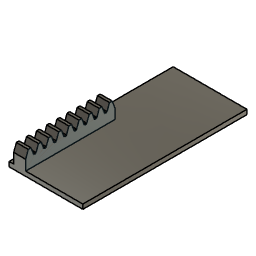
puerta mecatronica v1 (Autodesk Fusion 360 design; units mm, degrees)
Autodesk Fusion 360 part; units mm, degrees
sketch "Boceto1" plane through (0, 0, 0) normal (1, 0, 0) x (0, 1, 0)
  line L0 (0, 0) -> (1.5924, 4.375)
  line L1 (7.1092, 4.375) -> (8.7018, 0)
  line L2 (1.5924, 4.375) -> (2.8663, 7.875)
  line L3 (7.1092, 4.375) -> (5.8351, 7.875)
  line L4 (2.8663, 7.875) -> (5.8351, 7.875)
  line L5 (8.7018, 0) -> (0, 0)
  dimension "d8" = 4.375
  dimension "d9" = 3.5
  dimension "d10" = 3.5
  dimension "d11" = 4.375
  constraint coincident L0.start L5.end
  constraint parallel L0 L2
  constraint parallel L1 L3
  constraint horizontal L5
  measures "d8" vertical distance of L0.start L0.end
  measures "d9" vertical distance of L0.end L2.end
  measures "d10" vertical distance of L1.start L3.end
  measures "d11" vertical distance of L1.start L1.end
extrude "Extruir1" add sketch "Boceto1" along normal blind 13 makes body 1
pattern_linear "Patrón R1" count 9 spacing 11 along (0, -1, 0) of "Extruir1" makes body 2 makes body 3 makes body 4 makes body 5 makes body 6 makes body 7 makes body 8 makes body 9
sketch "Boceto2" plane through (13, 0, 0) normal (1, 0, 0) x (0, 1, 0)
  line L0 (8.7018, 0) -> (5.8351, 7.875)
  line L1 (5.8351, 7.875) -> (2.8663, 7.875)
  line L2 (2.8663, 7.875) -> (0, 0)
  line L3 (0, 0) -> (8.7018, 0)
  line L4 (-88, 0) -> (9, 0)
  line L5 (9, 0) -> (9, -16)
  line L6 (9, -16) -> (-88, -16)
  line L7 (-88, -16) -> (-88, 0)
  dimension "d18" = 16
  constraint horizontal L4
  constraint vertical L5
  constraint horizontal L6
  constraint vertical L7
  measures "d18" distance of L4.start L6.end
extrude "Extruir2" add sketch "Boceto2" against normal blind 13 contours L3 L4 L5 L6 L7 bodies 1 2 3 4 5 6 7 8 9
sketch "Boceto3" plane through (0, 0, 0) normal (-1, 0, 0) x (0, -1, 0)
  line L0 (71.1649, 7.875) -> (68.2982, 0)
  line L1 (68.2982, 0) -> (66, 0)
  line L2 (66, 0) -> (63.1337, 7.875)
  line L3 (63.1337, 7.875) -> (60.1649, 7.875)
  line L4 (60.1649, 7.875) -> (57.2982, 0)
  line L5 (57.2982, 0) -> (55, 0)
  line L6 (55, 0) -> (52.1337, 7.875)
  line L7 (52.1337, 7.875) -> (49.1649, 7.875)
  line L8 (49.1649, 7.875) -> (46.2982, 0)
  line L9 (46.2982, 0) -> (44, 0)
  line L10 (44, 0) -> (41.1337, 7.875)
  line L11 (41.1337, 7.875) -> (38.1649, 7.875)
  line L12 (38.1649, 7.875) -> (35.2982, 0)
  line L13 (35.2982, 0) -> (33, 0)
  line L14 (33, 0) -> (30.1337, 7.875)
  line L15 (30.1337, 7.875) -> (27.1649, 7.875)
  line L16 (27.1649, 7.875) -> (24.2982, 0)
  line L17 (24.2982, 0) -> (22, 0)
  line L18 (22, 0) -> (19.1337, 7.875)
  line L19 (19.1337, 7.875) -> (16.1649, 7.875)
  line L20 (16.1649, 7.875) -> (13.2982, 0)
  line L21 (13.2982, 0) -> (11, 0)
  line L22 (11, 0) -> (8.1337, 7.875)
  line L23 (8.1337, 7.875) -> (5.1649, 7.875)
  line L24 (5.1649, 7.875) -> (2.2982, 0)
  line L25 (2.2982, 0) -> (0, 0)
  line L26 (0, 0) -> (-2.8663, 7.875)
  line L27 (-2.8663, 7.875) -> (-5.8351, 7.875)
  line L28 (-5.8351, 7.875) -> (-8.7018, 0)
  line L29 (-8.7018, 0) -> (-9, 0)
  line L30 (-9, 0) -> (-9, -16)
  line L31 (-9, -16) -> (88, -16)
  line L32 (88, -16) -> (88, 0)
  line L33 (88, 0) -> (85.1337, 7.875)
  line L34 (85.1337, 7.875) -> (82.1649, 7.875)
  line L35 (82.1649, 7.875) -> (79.2982, 0)
  line L36 (79.2982, 0) -> (77, 0)
  line L37 (77, 0) -> (74.1337, 7.875)
  line L38 (74.1337, 7.875) -> (71.1649, 7.875)
  line L39 (-9, -16) -> (88, -16)
  line L40 (88, -16) -> (88, -11)
  line L41 (88, -11) -> (-9, -11)
  line L42 (-9, -11) -> (-9, -16)
  constraint horizontal L39
  constraint vertical L40
  constraint horizontal L41
  constraint vertical L42
  constraint coincident L32 L40.end
  constraint coincident L30.end L31.start
extrude "Extruir3" add sketch "Boceto3" along normal blind 5 contours L30 L31 L32 L39 L40 L41 L42 bodies 1
sketch "Boceto4" plane through (13, 0, 0) normal (1, 0, 0) x (0, 1, 0)
  line L0 (-68.2982, 0) -> (-71.1649, 7.875)
  line L1 (-71.1649, 7.875) -> (-74.1337, 7.875)
  line L2 (-74.1337, 7.875) -> (-77, 0)
  line L3 (-77, 0) -> (-79.2982, 0)
  line L4 (-79.2982, 0) -> (-82.1649, 7.875)
  line L5 (-82.1649, 7.875) -> (-85.1337, 7.875)
  line L6 (-85.1337, 7.875) -> (-88, 0)
  line L7 (-88, 0) -> (-88, -16)
  line L8 (-88, -16) -> (9, -16)
  line L9 (9, -16) -> (9, 0)
  line L10 (9, 0) -> (8.7018, 0)
  line L11 (8.7018, 0) -> (5.8351, 7.875)
  line L12 (5.8351, 7.875) -> (2.8663, 7.875)
  line L13 (2.8663, 7.875) -> (0, 0)
  line L14 (0, 0) -> (-2.2982, 0)
  line L15 (-2.2982, 0) -> (-5.1649, 7.875)
  line L16 (-5.1649, 7.875) -> (-8.1337, 7.875)
  line L17 (-8.1337, 7.875) -> (-11, 0)
  line L18 (-11, 0) -> (-13.2982, 0)
  line L19 (-13.2982, 0) -> (-16.1649, 7.875)
  line L20 (-16.1649, 7.875) -> (-19.1337, 7.875)
  line L21 (-19.1337, 7.875) -> (-22, 0)
  line L22 (-22, 0) -> (-24.2982, 0)
  line L23 (-24.2982, 0) -> (-27.1649, 7.875)
  line L24 (-27.1649, 7.875) -> (-30.1337, 7.875)
  line L25 (-30.1337, 7.875) -> (-33, 0)
  line L26 (-33, 0) -> (-35.2982, 0)
  line L27 (-35.2982, 0) -> (-38.1649, 7.875)
  line L28 (-38.1649, 7.875) -> (-41.1337, 7.875)
  line L29 (-41.1337, 7.875) -> (-44, 0)
  line L30 (-44, 0) -> (-46.2982, 0)
  line L31 (-46.2982, 0) -> (-49.1649, 7.875)
  line L32 (-49.1649, 7.875) -> (-52.1337, 7.875)
  line L33 (-52.1337, 7.875) -> (-55, 0)
  line L34 (-55, 0) -> (-57.2982, 0)
  line L35 (-57.2982, 0) -> (-60.1649, 7.875)
  line L36 (-60.1649, 7.875) -> (-63.1337, 7.875)
  line L37 (-63.1337, 7.875) -> (-66, 0)
  line L38 (-66, 0) -> (-68.2982, 0)
  line L39 (9, -16) -> (-88, -16)
  line L40 (-88, -16) -> (-88, -11)
  line L41 (-88, -11) -> (9, -11)
  line L42 (9, -11) -> (9, -16)
  constraint horizontal L39
  constraint vertical L40
  constraint horizontal L41
  constraint vertical L42
  constraint coincident L7 L40.end
  constraint coincident L8.end L9.start
extrude "Extruir4" add sketch "Boceto4" along normal blind 62 contours L7 L8 L9 L39 L40 L41 L42 bodies 1
sketch "Boceto5" plane through (13, 0, 0) normal (1, 0, 0) x (0, 1, 0)
  line L0 (-88, -11) -> (9, -11)
  line L1 (9, -11) -> (9, 0)
  line L2 (9, 0) -> (8.7018, 0)
  line L3 (8.7018, 0) -> (5.8351, 7.875)
  line L4 (5.8351, 7.875) -> (2.8663, 7.875)
  line L5 (2.8663, 7.875) -> (0, 0)
  line L6 (0, 0) -> (-2.2982, 0)
  line L7 (-2.2982, 0) -> (-5.1649, 7.875)
  line L8 (-5.1649, 7.875) -> (-8.1337, 7.875)
  line L9 (-8.1337, 7.875) -> (-11, 0)
  line L10 (-11, 0) -> (-13.2982, 0)
  line L11 (-13.2982, 0) -> (-16.1649, 7.875)
  line L12 (-16.1649, 7.875) -> (-19.1337, 7.875)
  line L13 (-19.1337, 7.875) -> (-22, 0)
  line L14 (-22, 0) -> (-24.2982, 0)
  line L15 (-24.2982, 0) -> (-27.1649, 7.875)
  line L16 (-27.1649, 7.875) -> (-30.1337, 7.875)
  line L17 (-30.1337, 7.875) -> (-33, 0)
  line L18 (-33, 0) -> (-35.2982, 0)
  line L19 (-35.2982, 0) -> (-38.1649, 7.875)
  line L20 (-38.1649, 7.875) -> (-41.1337, 7.875)
  line L21 (-41.1337, 7.875) -> (-44, 0)
  line L22 (-44, 0) -> (-46.2982, 0)
  line L23 (-46.2982, 0) -> (-49.1649, 7.875)
  line L24 (-49.1649, 7.875) -> (-52.1337, 7.875)
  line L25 (-52.1337, 7.875) -> (-55, 0)
  line L26 (-55, 0) -> (-57.2982, 0)
  line L27 (-57.2982, 0) -> (-60.1649, 7.875)
  line L28 (-60.1649, 7.875) -> (-63.1337, 7.875)
  line L29 (-63.1337, 7.875) -> (-66, 0)
  line L30 (-66, 0) -> (-68.2982, 0)
  line L31 (-68.2982, 0) -> (-71.1649, 7.875)
  line L32 (-71.1649, 7.875) -> (-74.1337, 7.875)
  line L33 (-74.1337, 7.875) -> (-77, 0)
  line L34 (-77, 0) -> (-79.2982, 0)
  line L35 (-79.2982, 0) -> (-82.1649, 7.875)
  line L36 (-82.1649, 7.875) -> (-85.1337, 7.875)
  line L37 (-85.1337, 7.875) -> (-88, 0)
  line L38 (-88, 0) -> (-88, -11)
sketch "Boceto6" plane through (0, 9, 0) normal (0, 1, 0) x (-1, 0, 0)
  line L0 (-13, 0) -> (-13, -11)
  line L1 (-13, -11) -> (-75, -11)
  line L2 (-75, -11) -> (-75, -16)
  line L3 (-75, -16) -> (5, -16)
  line L4 (5, -16) -> (5, -11)
  line L5 (5, -11) -> (0, -11)
  line L6 (0, -11) -> (0, 0)
  line L7 (0, 0) -> (-13, 0)
  line L8 (-75, -11) -> (5, -11)
  line L9 (5, -11) -> (5, -16)
  line L10 (5, -16) -> (-75, -16)
  line L11 (-75, -16) -> (-75, -11)
  constraint horizontal L8
  constraint vertical L9
  constraint horizontal L10
  constraint vertical L11
  constraint coincident L3.end L4.start
  constraint coincident L1.end L2.start
extrude "Extruir5" add sketch "Boceto6" along normal blind 81 contours L1 L2 L3 L4 L5 L8 L9 L10 L11 bodies 1
fillet "Empalme1" radius 1.05 17 edges at (6.5, -79.2982, 0) (6.5, -77, 0) (6.5, -68.2982, 0) (6.5, -66, 0) (6.5, -57.2982, 0) (6.5, -55, 0) (6.5, -46.2982, 0) (6.5, -44, 0) (6.5, -35.2982, 0) (6.5, -33, 0) (6.5, -24.2982, 0) (6.5, -22, 0) (6.5, -13.2982, 0) (6.5, -11, 0) (6.5, -2.2982, 0) (6.5, 0, 0) (6.5, 8.7018, 0) on bodies 1
